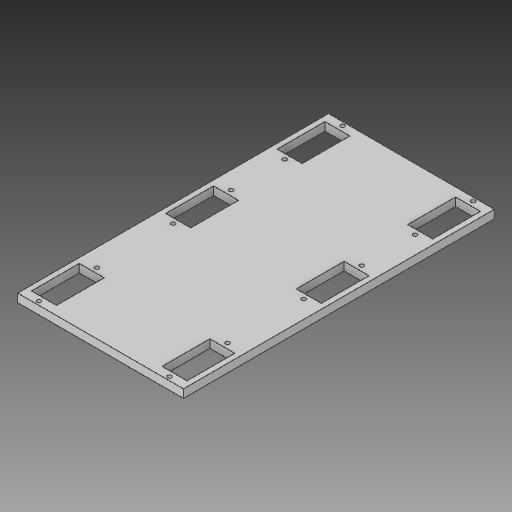
# Autodesk Inventor part: BODY_TOP
Saved by Autodesk Inventor 2017 (Build 210142000, 142)
## iProperties
Created: 2017-09-24
Part Number: BODY_TOP
Material: Generic
Document SubType Name: Modeling
Designer: Alexander Miller
Density: 1 g/cm^3
Appearance: Default
Author: Alexander Miller
Autodesk Inventor part; units mm, degrees
ref_plane "YZ Plane" through (0, 0, 0) normal (1, 0, 0) x (0, 1, 0)
ref_plane "XZ Plane" through (0, 0, 0) normal (0, 1, 0) x (-1, 0, 0)
ref_plane "XY Plane" through (0, 0, 0) normal (0, 0, 1) x (1, 0, 0)
sketch "Sketch1" plane through (0, 0, 0) normal (0, 1, 0) x (-1, 0, 0)
  line L0 (40, -75) -> (-40, -75)
  line L1 (-40, -75) -> (-40, 75)
  line L2 (-40, 75) -> (40, 75)
  line L3 (40, 75) -> (40, -75)
  point P0 (0, 0)
  point P1 (0, -75)
  point P2 (40, 0)
  dimension "d0" = 80
  dimension "d1" = 150
  constraints: 8 end point, 2 midpoint, 2 parallel, 1 horizontal, 1 horizontal alignment, 1 perpendicular, 1 vertical alignment
  measures "d0" distance of L0.start L0.end
  measures "d1" distance of L2.end L0.start
extrude "Extrusion1" add sketch "Sketch1" along normal blind 4
sketch "Sketch2" plane through (0, 4, 0) normal (0, 1, 0) x (1, 0, 0)
  line L0 (-37.5, 70.75) -> (-25.5, 70.75)
  line L1 (-25.5, 70.75) -> (-25.5, 47.75)
  line L2 (-25.5, 47.75) -> (-37.5, 47.75)
  line L3 (-37.5, 47.75) -> (-37.5, 70.75)
  line L4 (-37.5, 17) -> (-25.5, 17)
  line L5 (-25.5, 17) -> (-25.5, -6)
  line L6 (-25.5, -6) -> (-37.5, -6)
  line L7 (-37.5, -6) -> (-37.5, 17)
  line L8 (-37.5, -47.75) -> (-25.5, -47.75)
  line L9 (-25.5, -47.75) -> (-25.5, -70.75)
  line L10 (-25.5, -70.75) -> (-37.5, -70.75)
  line L11 (-37.5, -70.75) -> (-37.5, -47.75)
  line L12 (-40, 75) -> (-40, -75) projected
  line L13 (40, 75) -> (-40, 75) projected
  line L14 (-40, -75) -> (40, -75) projected
  circle A0 centre (-31.5, 0) radius 6 construction
  circle A1 centre (-31.5, 73.25) radius 1
  circle A2 centre (-31.5, 45.25) radius 1
  circle A3 centre (-31.5, 19.5) radius 1
  circle A4 centre (-31.5, -8.5) radius 1
  circle A5 centre (-31.5, -45.25) radius 1
  circle A6 centre (-31.5, -73.25) radius 1
  line L15 (0, 105) -> (0, -105) construction
  line L16 (37.5, 70.75) -> (25.5, 70.75)
  line L17 (25.5, 70.75) -> (25.5, 47.75)
  line L18 (25.5, 47.75) -> (37.5, 47.75)
  line L19 (37.5, 47.75) -> (37.5, 70.75)
  line L20 (37.5, 17) -> (25.5, 17)
  line L21 (25.5, 17) -> (25.5, -6)
  line L22 (25.5, -6) -> (37.5, -6)
  line L23 (37.5, -6) -> (37.5, 17)
  line L24 (37.5, -47.75) -> (25.5, -47.75)
  line L25 (25.5, -47.75) -> (25.5, -70.75)
  line L26 (25.5, -70.75) -> (37.5, -70.75)
  line L27 (37.5, -70.75) -> (37.5, -47.75)
  circle A7 centre (31.5, 73.25) radius 1
  circle A8 centre (31.5, 45.25) radius 1
  circle A9 centre (31.5, 19.5) radius 1
  circle A10 centre (31.5, -8.5) radius 1
  circle A11 centre (31.5, -45.25) radius 1
  circle A12 centre (31.5, -73.25) radius 1
  point P0 (0, 0)
  point P1 (-31.5, 47.75)
  point P2 (-31.5, 17)
  point P3 (-31.5, -6)
  point P4 (-31.5, -47.75)
  point P5 (-31.5, 70.75)
  point P6 (-31.5, -70.75)
  dimension "d4" = 2.5
  dimension "d5" = 4.25
  dimension "d6" = 23
  dimension "d7" = 12
  dimension "d8" = 4.25
  dimension "d9" = 2
  dimension "d10" = 1.5
  dimension "d11" = 1.5
  dimension "d12" = 1.5
  dimension "d13" = 1.5
  dimension "d14" = 1.5
  dimension "d15" = 1.5
  constraints: 48 end point, 18 symmetric about line, 13 centre point, 8 vertical alignment, 6 midpoint, 6 parallel, 5 equal radius, 3 equal length, 3 horizontal, 3 perpendicular, 3 tangent, 2 point on line, 1 horizontal alignment, 6 other
  measures "d4" distance between parallel lines of L3 L12
  measures "d5" distance between parallel lines of L13 L0
  measures "d6" distance of L2.end L0.start
  measures "d7" distance of L0.start L0.end
  measures "d8" distance between parallel lines of L14 L10
  measures "d9" diameter of A1
  measures "d10" distance edge to line of A1 L0
  measures "d11" distance edge to line of A2 L2
  measures "d12" distance edge to line of A3 L4
  measures "d13" distance edge to line of A4 L6
  measures "d14" distance edge to line of A5 L8
  measures "d15" distance edge to line of A6 L10
extrude "Extrusion2" cut sketch "Sketch2" against normal through all
equation "\"d0\" = body_B"
equation "\"d1\" = body_A"
equation "\"d2\" = body_C_Top"
equation "\"d4\" = 0.5 * body_C"
equation "\"d5\" = -0.5 * servo_A + 0.5 * servo_D"
equation "\"d6\" = servo_A"
equation "\"d7\" = servo_B"
equation "\"d8\" = d5"
equation "\"d9\" = servo_H"
equation "\"d10\" = servo_L"
equation "\"d11\" = d10"
equation "\"d12\" = d10"
equation "\"d13\" = d10"
equation "\"d14\" = d10"
equation "\"d15\" = d10"
equation "\"d16\" = body_C"
equation "\"body_B\" = 80"
equation "\"body_A\" = 150"
equation "\"body_C_Top\" = 4"
equation "\"body_C\" = 5"
equation "\"servo_A\" = 23"
equation "\"servo_D\" = 31.5"
equation "\"servo_B\" = 12"
equation "\"servo_H\" = 2"
equation "\"servo_L\" = 1.5"
body "Solid1"
